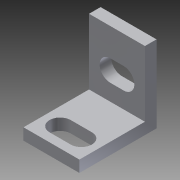
# Autodesk Inventor part: L bracket single
Saved by Autodesk Inventor 2014 SP1 (Build 180222100, 222)
## iProperties
Created: 2016-04-18
Part Number: L bracket single
Material: Generic
Document SubType Name: Modeling
Designer: Ben
Density: 1 g/cm^3
Appearance: Default
Author: Ben
Autodesk Inventor part; units mm, degrees
ref_plane "YZ Plane" through (0, 0, 0) normal (1, 0, 0) x (0, 1, 0)
ref_plane "XZ Plane" through (0, 0, 0) normal (0, 1, 0) x (-1, 0, 0)
ref_plane "XY Plane" through (0, 0, 0) normal (0, 0, 1) x (1, 0, 0)
sketch "Sketch1" plane through (0, 0, 0) normal (0, 0, 1) x (1, 0, 0)
  line L0 (-7.25, 10) -> (7.25, 10)
  line L1 (7.25, 10) -> (7.25, -10)
  line L2 (7.25, -10) -> (-7.25, -10)
  line L3 (-7.25, -10) -> (-7.25, 10)
  line L4 (0, 10) -> (0, -10) construction
  line L5 (-7.25, 0) -> (7.25, 0) construction
  line L6 (-1.75, 0) -> (1.75, 0) construction
  line L7 (-1.75, -2.75) -> (1.75, -2.75)
  line L8 (1.75, 2.75) -> (-1.75, 2.75)
  arc A0 (-1.75, 2.75) -> (-1.75, -2.75) centre (-1.75, 0) ccw
  arc A1 (1.75, -2.75) -> (1.75, 2.75) centre (1.75, 0) ccw
  point P0 (0, 0)
  point P1 (0, 0)
  dimension "d0" = 20
  dimension "d1" = 14.5
  dimension "d2" = 5.5
  dimension "d3" = 3.5
  dimension "d4" = 10
  constraints: 20 end point, 8 midpoint, 4 point on circle, 4 tangent, 3 parallel, 2 centre point, 2 perpendicular, 2 point on line, 1 horizontal
  measures "d0" distance of L2.end L0.start
  measures "d1" distance of L0.start L0.end
  measures "d2" diameter of A1
  measures "d3" distance of L6.end L6.start
  measures "d4" distance between parallel lines of L0 L5
extrude "Extrusion1" add sketch "Sketch1" along normal blind 3
sketch "Sketch2" plane through (0, 0, 3) normal (0, 0, 1) x (1, 0, 0)
  line L0 (7.25, -10) -> (7.25, 10) projected
  line L1 (-7.25, -10) -> (7.25, -10)
  line L2 (7.25, -10) -> (7.25, -7)
  line L3 (7.25, -7) -> (-7.25, -7)
  line L4 (-7.25, -7) -> (-7.25, -10)
  point P0 (0, 0)
  dimension "d7" = 3
  constraints: 8 end point, 2 parallel, 1 horizontal, 1 perpendicular, 1 point on line
  measures "d7" distance of L1.end L2.end
extrude "Extrusion2" add sketch "Sketch2" along normal blind 17
sketch "Sketch3" plane through (-7.25, -7, 3) normal (0, 1, 0) x (1, 0, 0)
  line L0 (0, 0) -> (0, -17) projected
  line L1 (14.5, -17) -> (0, -17) projected
  line L2 (14.5, 0) -> (14.5, -17) projected
  line L3 (0, -12) -> (14.5, -12) construction
  line L4 (4.5, -12) -> (10, -12) construction
  line L5 (4.5, -14.75) -> (10, -14.75)
  line L6 (10, -9.25) -> (4.5, -9.25)
  arc A0 (4.5, -9.25) -> (4.5, -14.75) centre (4.5, -12) ccw
  arc A1 (10, -14.75) -> (10, -9.25) centre (10, -12) ccw
  point P0 (7.25, 3)
  point P1 (7.25, -12)
  point P2 (7.25, -12)
  dimension "d10" = 5.5
  dimension "d11" = 5.5
  dimension "d12" = 5
  constraints: 10 end point, 4 point on circle, 4 point on line, 4 tangent, 2 centre point, 2 midpoint, 1 coincident, 1 parallel, 1 perpendicular
  measures "d10" diameter of A1
  measures "d11" distance of L4.end L4.start
  measures "d12" distance between parallel lines of L1 L3
extrude "Extrusion3" cut sketch "Sketch3" against normal up to surface (3 mm away)
ref_plane "Work Plane2" through (-5.5, -7, 15) normal (0, 0, 1) x (1, 0, 0)
body "Solid1"
